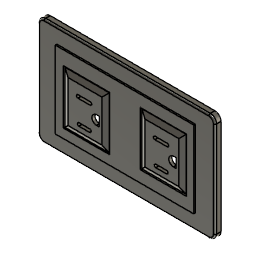
tomacorriente (Autodesk Fusion 360 design; units mm, degrees)
part number: 2026-03-28-22-37-53-552
Autodesk Fusion 360 part; units mm, degrees
sketch "Boceto1" plane through (0, 0, 0) normal (0, 1, 0) x (1, 0, 0)
  line L0 (303.7748, -214.9714) -> (196.7748, -214.9714)
  line L1 (192.7748, -218.9714) -> (192.7748, -284.9714)
  line L2 (196.7748, -284.9714) -> (303.7748, -284.9714)
  line L3 (307.7748, -280.9714) -> (307.7748, -218.9714)
  line L4 (307.7748, -214.9714) -> (192.7748, -284.9714) construction
  line L5 (192.7748, -214.9714) -> (307.7748, -284.9714) construction
  line L6 (192.7748, -280.9714) -> (192.7748, -248.4941)
  line L7 (192.7748, -248.4941) -> (217.7748, -248.4941)
  line L8 (307.7748, -250) -> (282.7748, -250)
  line L9 (282.7748, -250) -> (275.2748, -250)
  line L10 (260.2748, -232.5) -> (290.2748, -232.5)
  line L11 (290.2748, -232.5) -> (290.2748, -267.5)
  line L12 (290.2748, -267.5) -> (260.2748, -267.5)
  line L13 (260.2748, -267.5) -> (260.2748, -232.5)
  line L14 (260.2748, -232.5) -> (290.2748, -267.5) construction
  line L15 (290.2748, -232.5) -> (260.2748, -267.5) construction
  line L16 (217.7748, -248.4941) -> (225.2748, -248.4941)
  line L17 (240.2748, -230.9941) -> (210.2748, -230.9941)
  line L18 (210.2748, -230.9941) -> (210.2748, -265.9941)
  line L19 (210.2748, -265.9941) -> (240.2748, -265.9941)
  line L20 (240.2748, -265.9941) -> (240.2748, -230.9941)
  line L21 (240.2748, -230.9941) -> (210.2748, -265.9941) construction
  line L22 (210.2748, -230.9941) -> (240.2748, -265.9941) construction
  arc A0 (303.7748, -284.9714) -> (307.7748, -280.9714) centre (303.7748, -280.9714) ccw
  arc A1 (307.7748, -218.9714) -> (303.7748, -214.9714) centre (303.7748, -218.9714) ccw
  arc A2 (196.7748, -214.9714) -> (192.7748, -218.9714) centre (196.7748, -218.9714) ccw
  arc A3 (192.7748, -280.9714) -> (196.7748, -284.9714) centre (196.7748, -280.9714) ccw
  line L23 (225.2748, -265.9941) -> (225.2748, -257.4941)
  line L24 (225.2748, -230.9941) -> (225.2748, -239.4941)
  line L25 (229.4404, -254.9885) -> (221.4434, -254.9885)
  line L26 (221.4434, -256.9885) -> (229.4404, -256.9885)
  line L27 (163.1752, -254.9885) -> (212.7447, -256.9885) construction
  line L28 (212.7356, -254.9885) -> (222.7447, -256.9885) construction
  line L29 (229.0428, -239.5161) -> (222.0492, -239.5161)
  line L30 (222.0492, -241.5161) -> (229.0428, -241.5161)
  line L31 (225.2759, -239.5161) -> (225.3814, -241.5161) construction
  line L32 (225.3739, -239.5161) -> (234.3814, -241.5161) construction
  line L33 (225, -254.9885) -> (225, -241.5161)
  line L34 (225, -254.9885) -> (225, -241.5161)
  line L35 (240.2748, -248.4941) -> (232.7748, -248.4941)
  line L36 (233.5042, -245.6863) -> (235.2523, -245.6863)
  line L37 (235.2523, -245.6863) -> (235.2523, -251.6863)
  line L38 (235.2523, -251.6863) -> (233.5042, -251.6863)
  line L39 (230.5956, -245.6863) -> (235.2523, -251.6863) construction
  line L40 (235.2523, -245.6863) -> (229.9579, -251.6863) construction
  arc A4 (230.5042, -248.6975) -> (233.5042, -251.6863) centre (233.5042, -248.6863) ccw
  arc A5 (233.5042, -245.6863) -> (230.5042, -248.6975) centre (233.5042, -248.6863) ccw
  arc A6 (220.4434, -255.9921) -> (221.4434, -256.9885) centre (221.4434, -255.9885) ccw
  arc A7 (221.4434, -254.9885) -> (220.4434, -255.9921) centre (221.4434, -255.9885) ccw
  arc A8 (229.4404, -256.9885) -> (230.4404, -255.9849) centre (229.4404, -255.9885) ccw
  arc A9 (230.4404, -255.9849) -> (229.4404, -254.9885) centre (229.4404, -255.9885) ccw
  arc A10 (221.0492, -240.5205) -> (222.0492, -241.5161) centre (222.0492, -240.5161) ccw
  arc A11 (222.0492, -239.5161) -> (221.0492, -240.5205) centre (222.0492, -240.5161) ccw
  arc A12 (229.0428, -241.5161) -> (230.0427, -240.5117) centre (229.0428, -240.5161) ccw
  arc A13 (230.0427, -240.5117) -> (229.0428, -239.5161) centre (229.0428, -240.5161) ccw
  line L41 (270.7209, -257.1329) -> (278.7179, -257.1329)
  line L42 (278.7179, -255.1329) -> (270.7209, -255.1329)
  arc A14 (279.7179, -256.1293) -> (278.7179, -255.1329) centre (278.7179, -256.1329) ccw
  arc A15 (278.7179, -257.1329) -> (279.7179, -256.1293) centre (278.7179, -256.1329) ccw
  arc A16 (270.7209, -255.1329) -> (269.7209, -256.1365) centre (270.7209, -256.1329) ccw
  arc A17 (269.7209, -256.1365) -> (270.7209, -257.1329) centre (270.7209, -256.1329) ccw
  arc A18 (282.7817, -245.8307) -> (279.7817, -248.8419) centre (282.7817, -248.8307) ccw
  arc A19 (279.7817, -248.8419) -> (282.7817, -251.8307) centre (282.7817, -248.8307) ccw
  line L43 (284.5299, -251.8307) -> (282.7817, -251.8307)
  line L44 (284.5299, -245.8307) -> (284.5299, -251.8307)
  line L45 (282.7817, -245.8307) -> (284.5299, -245.8307)
  line L46 (278.3203, -239.6605) -> (271.3268, -239.6605)
  line L47 (271.3268, -241.6604) -> (278.3203, -241.6604)
  arc A20 (270.3268, -240.6649) -> (271.3268, -241.6604) centre (271.3268, -240.6604) ccw
  arc A21 (271.3268, -239.6605) -> (270.3268, -240.6649) centre (271.3268, -240.6605) ccw
  arc A22 (278.3203, -241.6604) -> (279.3203, -240.6561) centre (278.3203, -240.6604) ccw
  arc A23 (279.3203, -240.6561) -> (278.3203, -239.6605) centre (278.3203, -240.6605) ccw
  point P0 (250.2748, -249.9714)
  point P1 (275.2748, -250)
  point P2 (225.2748, -248.4941)
  point P3 (225.2748, -257.4941)
  point P4 (225.2748, -239.4941)
  point P5 (232.7748, -248.4941)
  dimension "d1" = 115
  dimension "d2" = 70
  dimension "d3" = 25
  dimension "d4" = 25
  dimension "d5" = 7.5
  dimension "d6" = 30
  dimension "d7" = 35
  dimension "d8" = 7.5
  dimension "d9" = 30
  dimension "d10" = 35
  dimension "d11" = 4
  dimension "d12" = 4
  dimension "d13" = 4
  dimension "d14" = 4
  dimension "d15" = 8.5
  dimension "d16" = 8.5
  dimension "d17" = 10
  dimension "d18" = 2
  dimension "d19" = 9
  dimension "d20" = 2
  dimension "d21" = 7.5
  dimension "d22" = 3
  dimension "d23" = 3
  dimension "d24" = 1
  dimension "d25" = 1
  dimension "d26" = 1
  dimension "d27" = 1
  dimension "d28" = 1
  dimension "d29" = 1
  dimension "d30" = 1
  dimension "d31" = 1
  dimension "d32" = 3
  dimension "d33" = 3
  dimension "d34" = 1
  dimension "d35" = 1
  dimension "d36" = 1
  dimension "d37" = 1
  dimension "d38" = 1
  dimension "d39" = 1
  dimension "d40" = 1
  dimension "d41" = 1
  constraint horizontal L0
  constraint perpendicular L0 L1
  constraint parallel L0 L2
  constraint parallel L1 L3
  constraint coincident L4 P0
  constraint coincident L5 P0
  constraint perpendicular L1 L7
  constraint perpendicular L3 L8
  constraint parallel L8 L9
  constraint horizontal L10
  constraint perpendicular L10 L11
  constraint parallel L10 L12
  constraint parallel L11 L13
  constraint coincident L14 P1
  constraint coincident L15 P1
  constraint coincident P1 L9.end
  constraint parallel L7 L16
  constraint horizontal L17
  constraint perpendicular L17 L18
  constraint parallel L17 L19
  constraint parallel L18 L20
  constraint coincident L21 P2
  constraint coincident L22 P2
  constraint coincident P2 L16.end
  constraint coincident L3 L8.start
  constraint coincident L5.end L2
  constraint coincident L5.end L3
  constraint tangent L2 A0
  constraint tangent L3 A0
  constraint coincident L4.start L0
  constraint coincident L4.start L3
  constraint tangent L0 A1
  constraint tangent L3 A1
  constraint coincident L1 L6.end
  constraint coincident L5.start L1
  constraint coincident L5.start L0
  constraint tangent L1 A2
  constraint tangent L0 A2
  constraint coincident L1.end L6
  constraint coincident L1.end L2
  constraint tangent L6 A3
  constraint tangent L2 A3
  constraint midpoint L19 L23.start
  constraint perpendicular L19 L23
  constraint midpoint L17 L24.start
  constraint perpendicular L17 L24
  constraint horizontal L25
  constraint parallel L25 L26
  constraint coincident L27 P3
  constraint coincident L28 P3
  constraint coincident P3 L23.end
  constraint horizontal L29
  constraint parallel L29 L30
  constraint coincident L31 P4
  constraint coincident L32 P4
  constraint coincident P4 L24.end
  constraint midpoint L20 L35.start
  constraint perpendicular L20 L35
  constraint horizontal L36
  constraint perpendicular L36 L37
  constraint parallel L36 L38
  constraint coincident L39 P5
  constraint coincident L40 P5
  constraint coincident P5 L35.end
  constraint coincident L40.end L38
  constraint tangent L38 A4
  constraint coincident L39.start L36
  constraint tangent L36 A5
  constraint coincident A4.start A5.end
  constraint coincident L27.end L26
  constraint tangent L26 A6
  constraint coincident L25 L33.start
  constraint coincident L28.start L25
  constraint tangent L25 A7
  constraint coincident A6.start A7.end
  constraint coincident L28.end L26
  constraint tangent L26 A8
  constraint coincident L27.start L25
  constraint tangent L25 A9
  constraint coincident A8.end A9.start
  constraint coincident L30 L33.end
  constraint coincident L31.end L30
  constraint tangent L30 A10
  constraint coincident L32.start L29
  constraint tangent L29 A11
  constraint coincident A10.start A11.end
  constraint coincident L32.end L30
  constraint tangent L30 A12
  constraint coincident L31.start L29
  constraint tangent L29 A13
  constraint coincident A12.end A13.start
  constraint horizontal L42
  constraint parallel L41 L42
  constraint horizontal L46
  constraint parallel L46 L47
  constraint horizontal L45
  constraint perpendicular L44 L45
  constraint parallel L43 L45
  constraint tangent A19 L43
  constraint tangent A18 L45
  constraint coincident A18.end A19.start
  constraint tangent L41 A17
  constraint tangent L42 A16
  constraint coincident A16.end A17.start
  constraint tangent L41 A15
  constraint tangent L42 A14
  constraint coincident A14.start A15.end
  constraint tangent L47 A20
  constraint tangent L46 A21
  constraint coincident A20.start A21.end
  constraint tangent L47 A22
  constraint tangent L46 A23
  constraint coincident A22.end A23.start
  measures "d1" distance of L1.end L5.end
  measures "d2" distance of L5.start L1.end
  measures "d3" distance of L6.end L7.end
  measures "d4" distance of L8.start L8.end
  measures "d5" distance of L8.end P1
  measures "d6" distance of L11.end L12.end
  measures "d7" distance of L10.end L11.end
  measures "d8" distance of L7.end P2
  measures "d9" distance of L18.end L19.end
  measures "d10" distance of L17.end L18.end
  measures "d11" radius of A0
  measures "d12" radius of A1
  measures "d13" radius of A2
  measures "d14" radius of A3
  measures "d15" distance of L23.start P3
  measures "d16" distance of L24.start P4
  measures "d17" distance of L27.end L28.end
  measures "d18" distance of L28.start L27.end
  measures "d19" distance of L31.end L32.end
  measures "d20" distance of L32.start L31.end
  measures "d21" distance of L35.start P5
  measures "d22" radius of A4
  measures "d23" radius of A5
  measures "d24" radius of A6
  measures "d25" radius of A7
  measures "d26" radius of A8
  measures "d27" radius of A9
  measures "d28" radius of A10
  measures "d29" radius of A11
  measures "d30" radius of A12
  measures "d31" radius of A13
  measures "d32" radius of A19
  measures "d33" radius of A18
  measures "d34" radius of A17
  measures "d35" radius of A16
  measures "d36" radius of A15
  measures "d37" radius of A14
  measures "d38" radius of A20
  measures "d39" radius of A21
  measures "d40" radius of A22
  measures "d41" radius of A23
extrude "Extruir1" add sketch "Boceto1" along normal blind 4 contours L0 L1 L2 L3 L6 A0 A1 A2 A3 makes body 1
extrude "Extruir2" add sketch "Boceto1" against normal blind 2 separate body contours L10 L11 L12 L13 makes body 2
chamfer "Chaflán1" distance 2 angle 45 2 edges at (275.2748, -2, 267.5) (260.2748, -2, 250) on bodies 2
chamfer "Chaflán2" distance 2 angle 45 2 edges at (290.2748, -2, 249) (276.2748, -2, 265.5) on bodies 2
chamfer "Chaflán3" distance 2 angle 45 2 edges at (262.2748, -2, 248) (275.2748, -2, 232.5) on bodies 2
chamfer "Chaflán4" distance 2 angle 45 2 edges at (288.2748, -2, 249) (276.2748, -2, 234.5) on bodies 2
copy_body "CopiarPegarCuerpos1" bodies 2 makes body 3
move_body "Desplazar1" bodies 3 to x (1, 0, 0) y (0, 1, 0) z (0, 0, 1) at (-49.966, 0, -1.6393)
fillet "Empalme1" radius 1 8 edges at (192.7748, 0, 249.9714) (193.9463, 0, 283.7998) (250.2748, 0, 284.9714) (306.6032, 0, 283.7998) (307.7748, 0, 249.9714) (306.6032, 0, 216.1429) (250.2748, 0, 214.9714) (193.9463, 0, 216.1429) on bodies 1
sketch "Boceto2" plane through (0, 0, 0) normal (0, -1, 0) x (1, 0, 0)
  line L0 (260.2748, 267.5) -> (290.2748, 267.5)
  line L1 (290.2748, 267.5) -> (290.2748, 232.5)
  line L2 (290.2748, 232.5) -> (260.2748, 232.5)
  line L3 (260.2748, 232.5) -> (260.2748, 267.5)
  line L4 (240.2748, 265.9941) -> (240.2748, 230.9941)
  line L5 (240.2748, 230.9941) -> (210.2748, 230.9941)
  line L6 (210.2748, 230.9941) -> (210.2748, 265.9941)
  line L7 (210.2748, 265.9941) -> (240.2748, 265.9941)
  line L8 (193.7748, 280.9714) -> (193.7748, 218.9714)
  arc A0 (193.7748, 218.9714) -> (196.7748, 215.9714) centre (196.7748, 218.9714) ccw
  line L9 (196.7748, 215.9714) -> (303.7748, 215.9714)
  arc A1 (303.7748, 215.9714) -> (306.7748, 218.9714) centre (303.7748, 218.9714) ccw
  line L10 (306.7748, 218.9714) -> (306.7748, 280.9714)
  arc A2 (306.7748, 280.9714) -> (303.7748, 283.9714) centre (303.7748, 280.9714) ccw
  line L11 (303.7748, 283.9714) -> (196.7748, 283.9714)
  arc A3 (196.7748, 283.9714) -> (193.7748, 280.9714) centre (196.7748, 280.9714) ccw
  line L12 (205, 275) -> (295, 275)
  line L13 (295, 275) -> (295, 225)
  line L14 (295, 225) -> (205, 225)
  line L15 (205, 225) -> (205, 275)
  line L16 (205, 275) -> (295, 225) construction
  line L17 (295, 275) -> (205, 225) construction
  point P0 (250, 250)
  constraint horizontal L12
  constraint perpendicular L12 L13
  constraint parallel L12 L14
  constraint parallel L13 L15
  constraint coincident L16 P0
  constraint coincident L17 P0
extrude "Extruir6" add sketch "Boceto2" along normal blind 1 contours L12 L13 L14 L15 bodies 1 3 2
